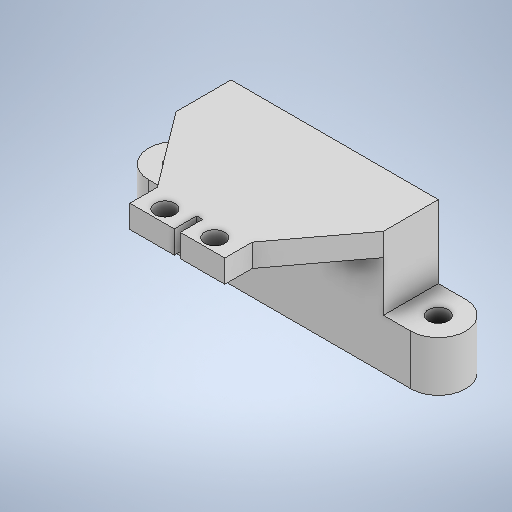
# Autodesk Inventor part: Servo holder long side
Saved by Autodesk Inventor 2025.1 (Build 291241000, 241)
## iProperties
Created: 2024-10-23
Part Number: Servo holder long side
Material: Generic
Document SubType Name: Modeling
Designer: m_kni
Density: 1 g/cm^3
Appearance: Default
Author: m_kni
Autodesk Inventor part; units mm, degrees
ref_plane "YZ Plane" through (0, 0, 0) normal (1, 0, 0) x (0, 1, 0)
ref_plane "XZ Plane" through (0, 0, 0) normal (0, 1, 0) x (-1, 0, 0)
ref_plane "XY Plane" through (0, 0, 0) normal (0, 0, 1) x (1, 0, 0)
sketch "Sketch1" plane through (0, 0, 0) normal (0, 1, 0) x (-1, 0, 0)
  circle A0 centre (-26.3449, -3.1424) radius 2
  arc A1 (-35.0949, -0.1424) -> (-17.5949, -0.1424) centre (-26.3449, -0.1424) ccw
  arc A2 (17.4051, -0.1424) -> (34.9051, -0.1424) centre (26.1551, -0.1424) ccw
  circle A3 centre (26.1551, -3.1424) radius 2
  circle A4 centre (-26.3449, -3.1424) radius 2
  circle A5 centre (26.1551, -3.1424) radius 2
  circle A6 centre (26.1551, -0.1424) radius 8.75
  circle A7 centre (-26.3449, -0.1424) radius 8.75
  line L0 (-35.0949, -0.1424) -> (-17.5949, -0.1424)
  line L1 (17.4051, -0.1424) -> (34.9051, -0.1424)
  circle A8 centre (-26.3449, -3.1424) radius 5.5
  circle A9 centre (26.1551, -3.1424) radius 5.5
  line L2 (-26.3449, -8.6424) -> (26.1551, -8.6424)
  line L3 (-26.3449, 2.3576) -> (26.1551, 2.3576)
  point P0 (0, 0)
  point P1 (-0.1898, -0.0949)
  dimension "d0" = 11
  dimension "d1" = 11
  constraints: 9 centre point, 8 end point, 8 point on circle, 6 coincident, 3 concentric, 2 tangent, 1 collinear, 1 horizontal, 1 horizontal alignment, 3 other
  measures "d0" diameter of A8
  measures "d1" diameter of A9
extrude "Extrusion1" add sketch "Sketch1" along normal blind 20 contours L2 A8 L0 A1 | A1 A7 L3 A6 A2 L2 | A7 L0 A8 L3 | A8 L0 | L0 A8 | A2 L1 A9 L2 | L3 A9 L1 A6 | A9 L1 | A9 L1 picked at (-18.8837, -1.0963) picked at (-20.7697, 1.0381) picked at (18.6638, -1.1758) picked at (20.5799, 1.0381)
sketch "Sketch2" plane through (0, 20, 0) normal (0, 1, 0) x (1, 0, 0)
  circle A0 centre (-26.1551, 3.1424) radius 2 projected
  circle A1 centre (26.3449, 3.1424) radius 2 projected
  circle A2 centre (-26.1551, 3.1424) radius 5.5
  circle A3 centre (26.3449, 3.1424) radius 5.5
  line L0 (26.3449, 8.6424) -> (-26.1551, 8.6424) projected
  line L1 (-20.6551, 8.6424) -> (-20.6551, -2.3576)
  line L2 (-26.1551, -2.3576) -> (26.3449, -2.3576) projected
  line L3 (20.8449, 8.6424) -> (20.8449, -2.3576)
  line L4 (-26.1551, 8.6424) -> (-20.6551, 8.6424)
  line L5 (-26.1551, -2.3576) -> (-20.6551, -2.3576)
  line L6 (20.8449, 8.6424) -> (26.3449, 8.6424)
  line L7 (20.8449, -2.3576) -> (26.3449, -2.3576)
  point P0 (0, 0)
  constraints: 12 end point, 3 tangent, 2 centre point, 2 coincident, 2 collinear, 2 parallel, 2 point on line, 2 vertical
extrude "Extrusion2" cut sketch "Sketch2" against normal blind 10 contours A2 | L1 L2 A2 | A2 L0 L1 | L0 A3 L3 | L3 A3 L2 | A3
sketch "Sketch4" plane through (0, 20, 0) normal (0, 1, 0) x (1, 0, 0)
  line L0 (20.8449, 8.6424) -> (-20.6551, 8.6424) projected
  line L1 (-20.6551, -2.3576) -> (20.8449, -2.3576) projected
  line L2 (-20.6551, 8.6424) -> (20.8449, 8.6424)
  line L3 (20.8449, 8.6424) -> (20.8449, -2.3576)
  line L4 (20.8449, -2.3576) -> (-20.6551, -2.3576)
  line L5 (-20.6551, -2.3576) -> (-20.6551, 8.6424)
  line L6 (-20.6551, -2.3576) -> (20.8449, -2.3576)
  line L7 (20.8449, -2.3576) -> (20.8449, -17.3636)
  line L8 (20.8449, -17.3636) -> (-20.6551, -17.3636)
  line L9 (-20.6551, -17.3636) -> (-20.6551, -2.3576)
  line L10 (9.5949, -22.8636) -> (-9.4051, -22.8636)
  line L11 (-9.4051, -22.8636) -> (-9.4051, -11.8636)
  line L12 (-9.4051, -11.8636) -> (9.5949, -11.8636)
  line L13 (9.5949, -11.8636) -> (9.5949, -22.8636)
  line L14 (9.5949, -22.8636) -> (-9.4051, -11.8636) construction
  line L15 (-9.4051, -22.8636) -> (9.5949, -11.8636) construction
  circle A0 centre (-4.9051, -20.3636) radius 2
  circle A1 centre (5.0949, -20.3636) radius 2
  point P0 (0, 0)
  point P1 (-9.4051, -17.3636)
  point P2 (9.5949, -17.3636)
  dimension "d27" = 19
  dimension "d28" = 11
  dimension "d29" = 4
  dimension "d30" = 3
  dimension "d31" = 4.5
  dimension "d32" = 4
  dimension "d33" = 3
  dimension "d34" = 4.5
  dimension "d37" = 20.506
  constraints: 28 end point, 6 parallel, 3 horizontal, 3 perpendicular, 2 centre point, 1 point on line
  measures "d27" distance of L11.end L12.end
  measures "d28" distance of L10.end L11.end
  measures "d29" diameter of A0
  measures "d30" distance from line of A0.centre L8
  measures "d31" distance from line of A0.centre L11
  measures "d32" diameter of A1
  measures "d33" distance from line of L8 A1.centre
  measures "d34" distance from line of L13 A1.centre
  measures "d37" distance between parallel lines of L1 L10
extrude "Extrusion5" add sketch "Sketch4" along normal blind 4.56
sketch "Sketch5" plane through (0, 24.56, 0) normal (0, 1, 0) x (1, 0, 0)
  line L0 (-9.4051, -22.8636) -> (9.5949, -22.8636) projected
  line L1 (9.5949, -17.3636) -> (20.8449, -17.3636) projected
  line L2 (-9.4051, -22.8636) -> (9.5949, -22.8636)
  line L3 (9.5949, -22.8636) -> (9.5949, -17.3636)
  line L4 (9.5949, -17.3636) -> (-9.4051, -17.3636)
  line L5 (-9.4051, -17.3636) -> (-9.4051, -22.8636)
  line L6 (-0.5051, -27.3636) -> (0.6949, -27.3636)
  line L7 (0.6949, -27.3636) -> (0.6949, -18.3636)
  line L8 (0.6949, -18.3636) -> (-0.5051, -18.3636)
  line L9 (-0.5051, -18.3636) -> (-0.5051, -27.3636)
  line L10 (-0.5051, -27.3636) -> (0.6949, -18.3636) construction
  line L11 (0.6949, -27.3636) -> (-0.5051, -18.3636) construction
  point P0 (0, 0)
  point P1 (0.0949, -22.8636)
  dimension "d41" = 1.2
  constraints: 20 end point, 4 parallel, 3 midpoint, 2 horizontal, 2 perpendicular
  measures "d41" distance of L8.end L7.end
extrude "Extrusion6" cut sketch "Sketch5" against normal blind 4.56 contours L9 L8 L7 L0 | L0 L7 L6 L9
sketch "Sketch6" plane through (0, 24.56, 0) normal (0, 1, 0) x (1, 0, 0)
  line L0 (26.3449, -2.3576) -> (20.8449, -2.3576) projected
  arc A0 (26.3449, -2.3576) -> (26.3449, 8.6424) centre (26.3449, 3.1424) ccw projected
  line L1 (20.8449, 8.6424) -> (26.3449, 8.6424) projected
  line L2 (20.8449, -2.3576) -> (20.8449, 8.6424) projected
  circle A1 centre (26.3449, 3.1424) radius 2 projected
  line L3 (-20.6551, -2.3576) -> (-26.1551, -2.3576) projected
  line L4 (-20.6551, 8.6424) -> (-20.6551, -2.3576) projected
  line L5 (-26.1551, 8.6424) -> (-20.6551, 8.6424) projected
  arc A2 (-26.1551, 8.6424) -> (-26.1551, -2.3576) centre (-26.1551, 3.1424) ccw projected
  circle A3 centre (-26.1551, 3.1424) radius 2 projected
  circle A4 centre (5.0949, -20.3636) radius 2 projected
  circle A5 centre (-4.9051, -20.3636) radius 2 projected
  line L6 (-0.5051, -22.8636) -> (-0.5051, -18.3636) projected
  line L7 (-0.5051, -18.3636) -> (0.6949, -18.3636) projected
  line L8 (0.6949, -18.3636) -> (0.6949, -22.8636) projected
  line L9 (0.6949, -22.8636) -> (9.5949, -22.8636) projected
  line L10 (9.5949, -22.8636) -> (9.5949, -17.3636) projected
  line L11 (9.5949, -17.3636) -> (20.8449, -17.3636) projected
  line L12 (20.8449, -17.3636) -> (20.8449, 8.6424) projected
  line L13 (20.8449, 8.6424) -> (-20.6551, 8.6424) projected
  line L14 (-20.6551, 8.6424) -> (-20.6551, -17.3636) projected
  line L15 (-20.6551, -17.3636) -> (-9.4051, -17.3636) projected
  line L16 (-9.4051, -17.3636) -> (-9.4051, -22.8636) projected
  line L17 (-9.4051, -22.8636) -> (-0.5051, -22.8636) projected
  line L18 (20.8449, -2.3576) -> (9.5949, -17.3636)
  line L19 (9.5949, -17.3636) -> (-9.4051, -17.3636)
  line L20 (20.8449, -17.3636) -> (20.8449, 8.6424) projected
  line L21 (-9.4051, -17.3636) -> (-20.6551, -2.3576)
  line L22 (-9.4051, -17.3636) -> (-20.6551, -17.3636)
  line L23 (-20.6551, -17.3636) -> (-20.6551, -2.3576)
  line L24 (20.8449, -17.3636) -> (9.5949, -17.3636)
  line L25 (20.8449, -17.3636) -> (20.8449, -2.3576)
  point P0 (0, 0)
  constraints: 14 end point, 3 collinear, 1 perpendicular
extrude "Extrusion7" cut sketch "Sketch6" against normal blind 4.56 contours L12 L11 L18 | L15 L14 L21
body "Solid1"
